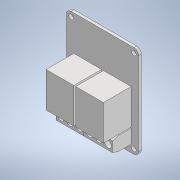
# Autodesk Inventor part: Dual Relay w Breakout Board
Saved by Autodesk Inventor 2020.2 (Build 242310000, 310)
## iProperties
Created: 2020-04-14
Part Number: Dual Relay w Breakout Board
Material: Generic
Document SubType Name: Modeling
Designer: Josiah
Density: 1 g/cm^3
Appearance: Default
Author: Josiah
Autodesk Inventor part; units mm, degrees
ref_plane "YZ Plane" through (0, 0, 0) normal (1, 0, 0) x (0, 1, 0)
ref_plane "XZ Plane" through (0, 0, 0) normal (0, 1, 0) x (-1, 0, 0)
ref_plane "XY Plane" through (0, 0, 0) normal (0, 0, 1) x (1, 0, 0)
sketch "Sketch1" plane through (0, 0, 0) normal (0, 0, 1) x (1, 0, 0)
  line L0 (-17, -25) -> (17, -25)
  line L1 (19.5, -22.5) -> (19.5, 22.5)
  line L2 (17, 25) -> (-17, 25)
  line L3 (-19.5, 22.5) -> (-19.5, -22.5)
  line L4 (19.5, -25) -> (-19.5, 25) construction
  circle A0 centre (16.95, -22.45) radius 1.25
  arc A1 (17, -25) -> (19.5, -22.5) centre (17, -22.5) ccw
  circle A2 centre (-16.95, -22.45) radius 1.25
  circle A3 centre (-16.95, 22.45) radius 1.25
  circle A4 centre (16.95, 22.45) radius 1.25
  arc A5 (19.5, 22.5) -> (17, 25) centre (17, 22.5) ccw
  arc A6 (-17, 25) -> (-19.5, 22.5) centre (-17, 22.5) ccw
  arc A7 (-19.5, -22.5) -> (-17, -25) centre (-17, -22.5) ccw
  point P0 (0, 0)
  point P1 (-19.5, -25)
  point P2 (19.5, 25)
  point P3 (0, 0)
  dimension "d0" = 50
  dimension "d1" = 39
  dimension "d2" = 2.5
  dimension "d3" = 2.55
  dimension "d4" = 2.55
  dimension "d5" = 2.5
  dimension "d6" = 2.5
  dimension "d7" = 2.5
  dimension "d8" = 2.5
  dimension "d9" = 2.55
  dimension "d10" = 2.55
  dimension "d11" = 2.55
  dimension "d12" = 2.55
  dimension "d13" = 2.55
  dimension "d14" = 2.55
  dimension "d15" = 2.5
  constraints: 10 end point, 8 centre point, 8 point on circle, 8 point on line, 8 tangent, 2 equal radius, 2 parallel, 1 coincident, 1 horizontal, 1 midpoint, 1 perpendicular
  measures "d0" distance of L4.end point (-19.5, -25)
  measures "d1" distance of point (19.5, 25) L4.end
  measures "d2" diameter of A0
  measures "d3" distance from line of A0.centre L0
  measures "d4" distance from line of A0.centre L1
  measures "d5" radius of A1
  measures "d6" diameter of A4
  measures "d7" diameter of A3
  measures "d8" diameter of A2
  measures "d9" distance from line of A2.centre L0
  measures "d10" distance from line of L3 A2.centre
  measures "d11" distance from line of L3 A3.centre
  measures "d12" distance from line of L2 A3.centre
  measures "d13" distance from line of L1 A4.centre
  measures "d14" distance from line of L2 A4.centre
  measures "d15" radius of A5
extrude "Extrusion1" add sketch "Sketch1" along normal blind 1.5
sketch "Sketch2" plane through (0, 0, 1.5) normal (0, 0, 1) x (1, 0, 0)
  line L0 (0.5, -13) -> (15.5, -13)
  line L1 (15.5, -13) -> (15.5, 6)
  line L2 (15.5, 6) -> (0.5, 6)
  line L3 (0.5, 6) -> (0.5, -13)
  line L4 (-15.5, -13) -> (-0.5, -13)
  line L5 (-0.5, -13) -> (-0.5, 6)
  line L6 (-0.5, 6) -> (-15.5, 6)
  line L7 (-15.5, 6) -> (-15.5, -13)
  line L8 (19.5, -22.5) -> (19.5, 22.5) projected
  line L9 (-19.5, 22.5) -> (-19.5, -22.5) projected
  line L10 (-17, -25) -> (17, -25) projected
  point P0 (0, 0)
  dimension "d18" = 15
  dimension "d19" = 19
  dimension "d22" = 16
  dimension "d27" = 4
  dimension "d28" = 39
  dimension "d29" = 12
  constraints: 16 end point, 2 horizontal, 2 parallel, 1 collinear, 1 perpendicular, 7 other
  measures "d18" distance of L1.end L2.end
  measures "d19" distance of L0.end L1.end
  measures "d22" distance of L0.start L4.start
  measures "d27" distance between parallel lines of L1 L8
  measures "d28" distance between parallel lines of L8 L9
  measures "d29" distance between parallel lines of L0 L10
extrude "Extrusion2" add sketch "Sketch2" along normal blind 15
sketch "Sketch3" plane through (0, 0, 1.5) normal (0, 0, 1) x (1, 0, 0)
  line L0 (0, -21) -> (-15, -21)
  line L1 (-15, -21) -> (-15, -13.5)
  line L2 (-15, -13.5) -> (0, -13.5)
  line L3 (0, -13.5) -> (0, -21)
  line L4 (-15.5, -13) -> (-0.5, -13) projected
  line L5 (-15.5, 6) -> (-15.5, -13) projected
  line L6 (15.5, -21) -> (0.5, -21)
  line L7 (0.5, -21) -> (0.5, -13.5)
  line L8 (0.5, -13.5) -> (15.5, -13.5)
  line L9 (15.5, -13.5) -> (15.5, -21)
  line L10 (0.5, -13) -> (15.5, -13) projected
  point P0 (0, 0)
  dimension "d32" = 15
  dimension "d33" = 7.5
  dimension "d34" = 0.5
  dimension "d35" = 0.5
  dimension "d36" = 15
  dimension "d37" = 7.5
  dimension "d38" = 0.5
  dimension "d39" = 0.5
  constraints: 16 end point, 4 parallel, 2 horizontal, 2 perpendicular
  measures "d32" distance of L1.end L2.end
  measures "d33" distance of L0.end L1.end
  measures "d34" distance between parallel lines of L4 L2
  measures "d35" distance between parallel lines of L5 L1
  measures "d36" distance of L7.end L8.end
  measures "d37" distance of L6.end L7.end
  measures "d38" distance between parallel lines of L3 L7
  measures "d39" distance between parallel lines of L8 L10
extrude "Extrusion3" add sketch "Sketch3" along normal blind 10
chamfer "Chamfer1" distance 1 distance2 3.5 1 edges at (8, -21, 11.5) measured on face at (10.5, -18.5, 11.5)
chamfer "Chamfer2" distance 1 distance2 3.5 1 edges at (8, -13.5, 11.5) measured on face at (10.5, -17.8333, 11.5)
chamfer "Chamfer3" distance 1 distance2 3.5 1 edges at (-7.5, -13.5, 11.5) measured on face at (-5, -18.5, 11.5)
chamfer "Chamfer4" distance 1 distance2 3.5 1 edges at (-7.5, -21, 11.5) measured on face at (-5, -18.8333, 11.5)
sketch "Sketch4" plane through (0, 0, 11.5) normal (0, 0, 1) x (1, 0, 0)
  line L0 (0.5, -14.5) -> (0.5, -20) projected
  line L1 (0, -20) -> (0, -14.5) projected
  line L2 (0.25, -35.642) -> (0.25, -29.5385) construction
  circle A0 centre (-12.5, -17.25) radius 1.75
  line L3 (-15, -14.5) -> (-15, -20) projected
  line L4 (-15, -14.5) -> (0, -14.5) projected
  line L5 (0, -20) -> (-15, -20) projected
  circle A1 centre (-7.5, -17.25) radius 1.75
  circle A2 centre (-2.5, -17.25) radius 1.75
  circle A3 centre (13, -17.25) radius 1.75
  circle A4 centre (8, -17.25) radius 1.75
  circle A5 centre (3, -17.25) radius 1.75
  point P0 (0, 0)
  dimension "d54" = 0.5
  dimension "d55" = 0.25
  dimension "d56" = 3.5
  dimension "d57" = 2.5
  dimension "d58" = 5.5
  dimension "d59" = 2.75
  dimension "d62" = 5
  constraints: 6 centre point, 3 symmetric about line, 2 end point, 1 horizontal, 1 vertical, 7 other
  measures "d54" distance between parallel lines of L0 L1
  measures "d55" distance between parallel lines of L1 L2
  measures "d56" diameter of A0
  measures "d57" distance from line of L3 A0.centre
  measures "d58" distance between parallel lines of L4 L5
  measures "d59" distance from line of A0.centre L5
  measures "d62" distance of A0.centre A1.centre
extrude "Extrusion4" cut sketch "Sketch4" against normal blind 3 contours A0 | A1 | A2 | A3 | A4 | A5
sketch "Sketch5" plane through (0.5, -21, 1.5) normal (0, -1, 0) x (1, 0, 0)
  line L0 (0.55, 5.5) -> (4.65, 5.5)
  line L1 (4.65, 5.5) -> (4.65, 1)
  line L2 (4.65, 1) -> (0.55, 1)
  line L3 (0.55, 1) -> (0.55, 5.5)
  line L4 (15, 10) -> (0, 10) projected
  line L5 (0, 0) -> (0, 6.5) projected
  line L6 (5.45, 1) -> (5.45, 5.5)
  line L7 (5.45, 5.5) -> (9.55, 5.5)
  line L8 (9.55, 1) -> (5.45, 1)
  line L9 (9.55, 5.5) -> (9.55, 1)
  line L10 (10.35, 1) -> (10.35, 5.5)
  line L11 (10.35, 5.5) -> (14.45, 5.5)
  line L12 (14.45, 1) -> (10.35, 1)
  line L13 (14.45, 5.5) -> (14.45, 1)
  line L14 (15, 0) -> (15, 6.5) projected
  line L15 (-0.5, 0) -> (-0.5, 6.5) projected
  line L16 (-0.25, -5.4551) -> (-0.25, -7.5555) construction
  line L17 (-1.05, 5.5) -> (-5.15, 5.5)
  line L18 (-5.15, 5.5) -> (-5.15, 1)
  line L19 (-5.15, 1) -> (-1.05, 1)
  line L20 (-1.05, 1) -> (-1.05, 5.5)
  line L21 (-5.95, 1) -> (-5.95, 5.5)
  line L22 (-5.95, 5.5) -> (-10.05, 5.5)
  line L23 (-10.05, 1) -> (-5.95, 1)
  line L24 (-10.05, 5.5) -> (-10.05, 1)
  line L25 (-10.85, 1) -> (-10.85, 5.5)
  line L26 (-10.85, 5.5) -> (-14.95, 5.5)
  line L27 (-14.95, 1) -> (-10.85, 1)
  line L28 (-14.95, 5.5) -> (-14.95, 1)
  point P0 (-0.5, -1.5)
  dimension "d71" = 4.1
  dimension "d72" = 4.5
  dimension "d73" = 4.5
  dimension "d74" = 0.55
  dimension "d77" = 4.9
  dimension "d85" = 0.5
  dimension "d86" = 0.25
  constraints: 50 end point, 12 symmetric about line, 2 horizontal, 2 parallel, 1 perpendicular, 1 vertical, 16 other
  measures "d71" distance of L0.start L0.end
  measures "d72" distance of L0.end L1.end
  measures "d73" distance between parallel lines of L0 L4
  measures "d74" distance between parallel lines of L5 L3
  measures "d77" distance of L2.end L6.start
  measures "d85" distance between parallel lines of L5 L15
  measures "d86" distance between parallel lines of L16 L5
extrude "Extrusion5" cut sketch "Sketch5" against normal blind 3
equation "\"d4\" = d3"
equation "\"d5\" = d2"
equation "\"d6\" = d2"
equation "\"d7\" = d2"
equation "\"d8\" = d2"
equation "\"d9\" = d3"
equation "\"d10\" = d3"
equation "\"d11\" = d3"
equation "\"d12\" = d3"
equation "\"d13\" = d3"
equation "\"d14\" = d3"
equation "\"d15\" = d2"
equation "\"d27\" = -0.5 * d22 + 0.5 * d28 - 0.5 * d18"
equation "\"d39\" = d34"
equation "\"d55\" = 0.5 * d54"
equation "\"d59\" = 0.5 * d58"
equation "\"d86\" = 0.5 * d85"
body "Solid1"
